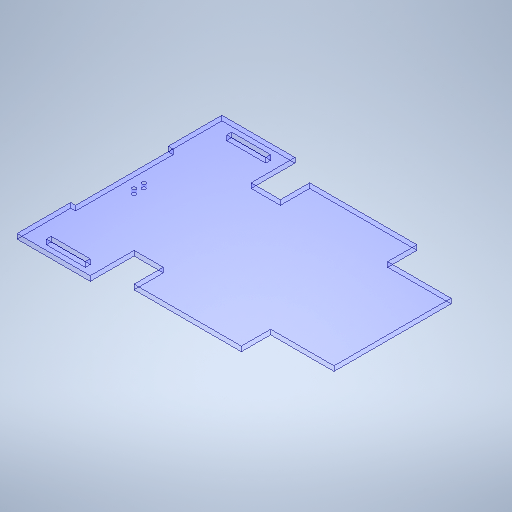
# Autodesk Inventor part: hood
Saved by Autodesk Inventor 2025.3 (Build 293356030, 356C)
## iProperties
Created: 2026-06-26
Part Number: hood
Material: Generic
Document SubType Name: Modeling
Designer: user
Density: 1 g/cm^3
Appearance: Blue
Author: user
Autodesk Inventor part; units mm, degrees
ref_plane "YZ Plane" through (0, 0, 0) normal (1, 0, 0) x (0, 1, 0)
ref_plane "XZ Plane" through (0, 0, 0) normal (0, 1, 0) x (-1, 0, 0)
ref_plane "XY Plane" through (0, 0, 0) normal (0, 0, 1) x (1, 0, 0)
sketch "Sketch1" plane through (0, 0, 0) normal (0, 1, 0) x (-1, 0, 0)
  line L0 (0, 0) -> (-75, 0)
  line L1 (-75, 0) -> (-75, -210)
  line L2 (-75, -210) -> (0, -210)
  line L3 (0, -210) -> (0, 0)
  line L4 (-20, -10) -> (-60, -10)
  line L5 (-60, -10) -> (-60, -15)
  line L6 (-60, -15) -> (-20, -15)
  line L7 (-20, -15) -> (-20, -10)
  line L8 (-75, -105) -> (0, -105) construction
  line L9 (-20, -200) -> (-60, -200)
  line L10 (-60, -200) -> (-60, -195)
  line L11 (-60, -195) -> (-20, -195)
  line L12 (-20, -195) -> (-20, -200)
  line L13 (-75, -45) -> (-280, -45)
  line L14 (-280, -45) -> (-280, -165)
  line L15 (-280, -165) -> (-75, -165)
  line L16 (-75, -165) -> (-75, -45)
  line L17 (0, -55) -> (-5, -55)
  line L18 (-5, -55) -> (-5, -155)
  line L19 (-5, -155) -> (0, -155)
  line L20 (0, -155) -> (0, -55)
  line L21 (-105, -45) -> (-215, -45)
  line L22 (-215, -45) -> (-215, -15)
  line L23 (-215, -15) -> (-105, -15)
  line L24 (-105, -15) -> (-105, -45)
  line L25 (-105, -165) -> (-215, -165)
  line L26 (-215, -165) -> (-215, -195)
  line L27 (-215, -195) -> (-105, -195)
  line L28 (-105, -195) -> (-105, -165)
  point P0 (-75, -165)
  point P1 (0, -155)
  dimension "d0" = 75
  dimension "d2" = 40
  dimension "d3" = 5
  dimension "d11" = 20
  dimension "d12" = 5
  dimension "d13" = 100
  dimension "d15" = 110
  dimension "d16" = 30
  dimension "d17" = 10
  dimension "d19" = 190
  dimension "d21" = 30
  dimension "d22" = 30
  dimension "d23" = 50
  dimension "d25" = 30
  dimension "d26" = 110
  dimension "d27" = 120
  dimension "d28" = 45
  dimension "d29" = 205
  constraints: 58 end point, 12 parallel, 6 horizontal, 6 perpendicular, 4 point on line, 4 symmetric about line, 2 midpoint
  measures "d0" distance of L2.end L1.end
  measures "d2" distance of L6.end L5.end
  measures "d3" distance of L5.end L4.end
  measures "d11" distance between parallel lines of L12 L3
  measures "d12" distance of L19.end L18.end
  measures "d13" distance of L18.end L17.end
  measures "d15" distance of L22.end L23.end
  measures "d16" distance between parallel lines of L24 L1
  measures "d17" distance between parallel lines of L0 L4
  measures "d19" distance between parallel lines of L4 L9
  measures "d21" distance between parallel lines of L25 L27
  measures "d22" distance between parallel lines of L21 L23
  measures "d23" distance between parallel lines of L8 L19
  measures "d25" distance between parallel lines of L1 L28
  measures "d26" distance between parallel lines of L26 L28
  measures "d27" distance between parallel lines of L13 L15
  measures "d28" distance between parallel lines of L15 L2
  measures "d29" distance between parallel lines of L14 L16
extrude "Extrusion1" add sketch "Sketch1" along normal blind 5 contours L3 L17 L18 L19 L2 L1 L0 | L1 L15 L14 L13 | L13 L22 L23 L24 | L28 L27 L26 L15
sketch "Sketch2" plane through (0, 5, 0) normal (0, 1, 0) x (1, 0, 0)
  line L0 (5, 155) -> (5, 55) projected
  line L1 (0, 155) -> (5, 155) projected
  point P0 (0, 0)
  point P1 (20, 100)
  point P2 (20, 110)
  dimension "d37" = 10
  dimension "d38" = 15
  dimension "d39" = 15
  dimension "d40" = 45
  measures "d37" distance of point (20, 100) point (20, 110)
  measures "d38" distance from line of L0 point (20, 110)
  measures "d39" distance from line of L0 point (20, 100)
  measures "d40" distance from line of point (20, 110) L1
hole "Hole1" at (20, 5, -100) at (20, 5, -110) direction (0, -1, 0) diameter 4 end through all
body "Solid1"
